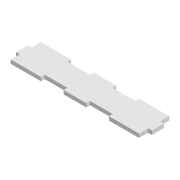
# Autodesk Inventor part: Superior 1
Saved by Autodesk Inventor 2022 (Build 260153000, 153)
## iProperties
Created: 2022-06-21
Part Number: Superior 1
Material: Generic
Document SubType Name: Modeling
Designer: ADMIN
Density: 1 g/cm^3
Appearance: Default
Author: ADMIN
Autodesk Inventor part; units mm, degrees
ref_plane "YZ Plane" through (0, 0, 0) normal (1, 0, 0) x (0, 1, 0)
ref_plane "XZ Plane" through (0, 0, 0) normal (0, 1, 0) x (-1, 0, 0)
ref_plane "XY Plane" through (0, 0, 0) normal (0, 0, 1) x (1, 0, 0)
sketch "Sketch1" plane through (0, 0, 0) normal (0, 1, 0) x (-1, 0, 0)
  line L0 (10.3774, 19.343) -> (-159.6226, 19.343)
  line L1 (-159.6226, 19.343) -> (-159.6226, -20.657)
  line L2 (-159.6226, -20.657) -> (10.3774, -20.657)
  line L3 (10.3774, -20.657) -> (10.3774, 19.343)
  line L4 (10.3774, 7.343) -> (15.3774, 7.343)
  line L5 (15.3774, 7.343) -> (15.3774, -8.657)
  line L6 (15.3774, -8.657) -> (10.3774, -8.657)
  line L7 (10.3774, -8.657) -> (10.3774, 7.343)
  line L8 (-159.6226, 7.343) -> (-164.6226, 7.343)
  line L9 (-164.6226, 7.343) -> (-164.6226, -8.657)
  line L10 (-164.6226, -8.657) -> (-159.6226, -8.657)
  line L11 (-159.6226, -8.657) -> (-159.6226, 7.343)
  line L12 (-119.6226, -20.657) -> (-89.6226, -20.657)
  line L13 (-89.6226, -20.657) -> (-89.6226, -15.657)
  line L14 (-89.6226, -15.657) -> (-119.6226, -15.657)
  line L15 (-119.6226, -15.657) -> (-119.6226, -20.657)
  line L16 (-59.6226, -20.657) -> (-29.6226, -20.657)
  line L17 (-29.6226, -20.657) -> (-29.6226, -15.657)
  line L18 (-29.6226, -15.657) -> (-59.6226, -15.657)
  line L19 (-59.6226, -15.657) -> (-59.6226, -20.657)
  line L20 (-159.6226, -0.657) -> (10.3774, -0.657) construction
  line L21 (-74.6226, 19.343) -> (-74.6226, -20.657) construction
  line L22 (-89.6226, 19.343) -> (-89.6226, 14.343)
  line L23 (-89.6226, 14.343) -> (-119.6226, 14.343)
  line L24 (-119.6226, 14.343) -> (-119.6226, 19.343)
  line L25 (-29.6226, 19.343) -> (-29.6226, 14.343)
  line L26 (-29.6226, 14.343) -> (-59.6226, 14.343)
  line L27 (-59.6226, 14.343) -> (-59.6226, 19.343)
  line L28 (-74.6226, -20.657) -> (-74.6226, 19.343) construction
  point P0 (0, 0)
  point P1 (10.3774, -8.657)
  point P2 (-159.6226, -8.657)
  point P3 (-89.6226, -20.657)
  point P4 (-29.6226, -20.657)
  point P5 (-29.6226, 19.343)
  point P6 (-59.6226, 19.343)
  point P7 (-89.6226, 19.343)
  point P8 (-119.6226, 19.343)
  dimension "d0" = 170
  dimension "d1" = 40
  dimension "d2" = 5
  dimension "d3" = 16
  dimension "d4" = 12
  dimension "d5" = 5
  dimension "d6" = 16
  dimension "d7" = 12
  dimension "d17" = 30
  dimension "d18" = 5
  dimension "d19" = 30
  dimension "d20" = 30
  dimension "d21" = 15
  constraints: 58 end point, 10 parallel, 10 symmetric about line, 6 perpendicular, 5 horizontal, 5 point on line, 3 midpoint
  measures "d0" distance of L2.end L1.end
  measures "d1" distance of L2.end L0.start
  measures "d2" distance of L5.end L6.end
  measures "d3" distance of L4.end L5.end
  measures "d4" distance between parallel lines of L4 L0
  measures "d5" distance of L10.end L9.end
  measures "d6" distance of L9.end L8.end
  measures "d7" distance between parallel lines of L0 L8
  measures "d17" distance of L14.end L13.end
  measures "d18" distance of L14.end L12.start
  measures "d19" distance of L18.end L17.end
  measures "d20" distance between parallel lines of L13 L19
  measures "d21" distance between parallel lines of L21 L13
extrude "Extrusion1" add sketch "Sketch1" along normal blind 5 contours L3 L2 L17 L18 L19 L13 L14 L15 L1 L0 L24 L23 L22 L27 L26 L25 | L4 L5 L6 L3 | L1 L10 L9 L8
equation "\"d3\" = d6"
equation "\"d7\" = d4"
body "Solid1"
